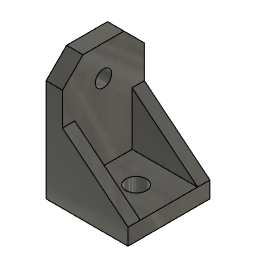
2040 Drybox Draw Brackets (Autodesk Fusion 360 design; units mm, degrees)
Autodesk Fusion 360 part; units mm, degrees
sketch "Sketch1" plane through (0, 0, 0) normal (0, 1, 0) x (1, 0, 0)
  line L0 (0, 0) -> (-4, 0)
  line L1 (-4, 0) -> (-4, -30)
  line L2 (-4, -30) -> (0, -30)
  line L3 (0, -30) -> (0, 0)
  line L4 (-4, 0) -> (16, 0)
  line L5 (16, 0) -> (16, -4)
  line L6 (16, -4) -> (-4, -4)
  line L7 (-4, -4) -> (-4, 0)
  dimension "d1" = 4
  dimension "d2" = 30
  dimension "d3" = 20
  dimension "d4" = 4
  constraint horizontal L0
  constraint vertical L1
  constraint horizontal L2
  constraint vertical L3
  constraint coincident L0.start L3.end
  constraint horizontal L4
  constraint vertical L5
  constraint horizontal L6
  constraint vertical L7
  measures "d1" distance of L0.start L0.end
  measures "d2" distance of L0.start L2.end
  measures "d3" distance of L0.end L4.end
  measures "d4" distance of L0.end L6.end
extrude "Extrude1" add sketch "Sketch1" along normal blind 20
sketch "Sketch2" plane through (0, 0, 0) normal (0, -1, 0) x (1, 0, 0)
  line L0 (0, 30) -> (-4, 30)
  line L1 (-4, 30) -> (-4, 0)
  line L2 (-4, 0) -> (16, 0)
  line L3 (16, 0) -> (16, 4)
  line L4 (16, 4) -> (0, 4)
  line L5 (0, 4) -> (0, 30)
  line L6 (0, 30) -> (16, 4)
  line L7 (16, 4) -> (0, 17)
  constraint coincident L0.start L5.end
  constraint coincident L3.end L4.start
  constraint midpoint L5 L7.end
extrude "Extrude2" add sketch "Sketch2" against normal blind 3 contours L4 L5 L7
extrude "Extrude3" add sketch "Sketch2" along normal blind 3 from surface at -20 contours L4 L5 L7
sketch "Sketch3" plane through (0, 0, 4) normal (0, 0, 1) x (-1, 0, 0)
  line L0 (-16, -17) -> (0, -17)
  line L1 (0, -17) -> (0, -3)
  line L2 (0, -3) -> (-16, -3)
  line L3 (-16, -3) -> (-16, -17)
  line L4 (-8, -17) -> (-8, -10)
  line L5 (-8, -10) -> (-16, -10)
  point P0 (-8, -13.5)
  point P1 (-8, -6.5)
  constraint midpoint L0 L4.start
  constraint perpendicular L0 L4
  constraint perpendicular L3 L5
  constraint midpoint L3 L5.end
  constraint midpoint L4 P0
  constraint symmetric L5 P0 P1
hole "Hole1" at (8, 10, 4) direction (0, 0, -1) diameter 5 depth 16 tip angle 118
hole "Hole2" at (-4, 10, 22.5) direction (1, 0, 0) diameter 4 depth 20 tip angle 118
chamfer "Chamfer1" distance 5 angle 45 2 edges at (-2, 0, 30) (-2, 20, 30)
